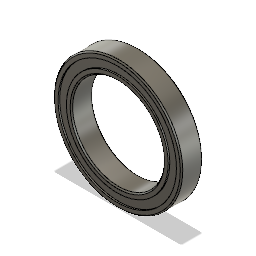
assembly (Autodesk Fusion 360 archive; units mm, degrees)
design "Bearing 42x30x7"
Autodesk Fusion 360 part; units mm, degrees
sketch "Sketch1" plane through (0, 0, 0) normal (0, 1, 0) x (1, 0, 0)
  line L0 (15, 0) -> (15, 3.5)
  line L1 (15, 3.5) -> (16.65, 3.5)
  line L2 (16.65, 3.5) -> (16.65, 3)
  line L3 (16.65, 3) -> (19.35, 3)
  line L4 (19.35, 3) -> (19.35, 3.5)
  line L5 (19.35, 3.5) -> (21, 3.5)
  line L6 (21, 3.5) -> (21, 0)
  line L7 (0, 0) -> (-6, 0) construction
  line L8 (15, 0) -> (15, -3.5)
  line L9 (16.65, -3) -> (19.35, -3)
  line L10 (19.35, -3) -> (19.35, -3.5)
  line L11 (16.65, -3.5) -> (16.65, -3)
  line L12 (15, -3.5) -> (16.65, -3.5)
  line L13 (21, -3.5) -> (21, 0)
  line L14 (19.35, -3.5) -> (21, -3.5)
  line L15 (0, 0) -> (0, 9) construction
  dimension "d3" = 3.5
  dimension "d4" = 3.5
  dimension "d5" = 15
  dimension "d6" = 21
  dimension "d7" = 2.7
  dimension "d8" = 3
  constraint vertical L0
  constraint perpendicular L0 L1
  constraint perpendicular L1 L2
  constraint perpendicular L0 L3
  constraint perpendicular L3 L4
  constraint perpendicular L4 L5
  constraint perpendicular L5 L6
  constraint coincident L7.start L15.start
  constraint parallel L3 L7
  constraint symmetric L0.start L7 L8.start
  constraint symmetric L0.end L7 L8.end
  constraint symmetric L1.end L7 L11.start
  constraint symmetric L2.end L7 L9.start
  constraint symmetric L3.end L7 L9.end
  constraint symmetric L4.end L7 L10.end
  constraint symmetric L5.end L7 L13.start
  constraint symmetric L6.end L7 L13.end
  constraint equal L1 L5
  constraint perpendicular L7 L15
  measures "d3" distance of L7.start L5
  measures "d4" distance of L7.start L1
  measures "d5" distance of L7.start L0
  measures "d6" distance of L7.start L6
  measures "d7" distance of L2.end L3.end
  measures "d8" distance of L7.start L3
revolve "Revolve1" add sketch "Sketch1" angle 360 about axis through (0, 0, 0) along (0, 0, -1)
chamfer "Chamfer1" distance 0.4 angle 45 4 edges at (-19.5789, -7.5939, -3.5) (-13.9849, -5.4242, -3.5) (-19.5789, -7.5939, 3.5) (-13.9849, -5.4242, 3.5)

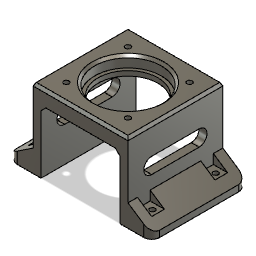
design "bearing_support"
Autodesk Fusion 360 part; units mm, degrees
sketch "Sketch1" plane through (0, 0, 0) normal (0, 0, 1) x (1, 0, 0)
  line L0 (-45, -42) -> (-45, -38)
  line L1 (-45, -38) -> (-30, -38)
  line L2 (-30, -38) -> (-30, 8)
  line L3 (-30, 8) -> (30, 8)
  line L4 (30, 8) -> (30, -38)
  line L5 (30, -38) -> (45, -38)
  line L6 (45, -38) -> (45, -42)
  line L7 (45, -42) -> (25, -42)
  line L8 (25, -42) -> (25, -2)
  line L9 (25, -2) -> (-25, -2)
  line L10 (-25, -2) -> (-25, -42)
  line L11 (-25, -42) -> (-45, -42)
  dimension "d1" = 60
  dimension "d2" = 30
  dimension "d3" = 4
  dimension "d4" = 4
  dimension "d5" = 5
  dimension "d6" = 5
  dimension "d7" = 10
  dimension "d8" = 15
  dimension "d9" = 15
  dimension "d24" = 46
  dimension "d25" = 46
  constraint vertical L0
  constraint perpendicular L0 L1
  constraint perpendicular L1 L2
  constraint perpendicular L2 L3
  constraint perpendicular L3 L4
  constraint perpendicular L4 L5
  constraint perpendicular L5 L6
  constraint perpendicular L6 L7
  constraint perpendicular L7 L8
  constraint perpendicular L8 L9
  constraint perpendicular L9 L10
  constraint perpendicular L0 L11
  measures "d1" distance of L2.end L3.end
  measures "d2" distance of origin L4
  measures "d3" distance of L5.end L6.end
  measures "d4" distance of L0.start L0.end
  measures "d5" distance of L4 L8
  measures "d6" distance of L2 L10
  measures "d7" distance of L3 L9
  measures "d8" distance of L4.end L5.end
  measures "d9" distance of L0.end L1.end
  measures "d24" distance of L3.end L4.end
  measures "d25" distance of L1.end L2.end
extrude "Extrude1" add sketch "Sketch1" along normal blind 60
sketch "Sketch2" plane through (0, 8, 0) normal (0, 1, 0) x (-1, 0, 0)
  line L0 (-30, 0) -> (30, 0)
  line L1 (30, 0) -> (30, 60)
  line L2 (30, 60) -> (-30, 60)
  line L3 (-30, 60) -> (-30, 0)
  circle A0 centre (0, 30) radius 21.1
  dimension "d14" = 42.2
  dimension "d15" = 30
  dimension "d16" = 30
  measures "d14" diameter of A0
  measures "d15" distance of L0 A0.centre
  measures "d16" distance of L3 A0.centre
extrude "Extrude2" cut sketch "Sketch2" against normal blind 7 contours A0
sketch "Sketch3" plane through (0, 1, 0) normal (0, 1, 0) x (-1, 0, 0)
  circle A0 centre (0, 30) radius 21.1
  circle A1 centre (0, 30) radius 19
  dimension "d20" = 38
  constraint concentric A0 A1
  measures "d20" diameter of A1
extrude "Extrude3" cut sketch "Sketch3" against normal up to surface (3 mm away) contours A1
chamfer "Chamfer1" distance 10 distance2 15 1 edges at (-30, -38, 30) measured on face at (-30, -22.6667, 40)
chamfer "Chamfer2" distance 15 distance2 10 1 edges at (30, -38, 30) measured on face at (35, -38, 20)
chamfer "Chamfer3" distance 1.5 angle 45 1 edges at (19.6721, 8, 37.6301)
chamfer "Chamfer4" distance 2 distance2 1 2 edges at (0, 8, 0) (0, 8, 60) measured on face at (33.3323, -36.0007, 0) measured on face at (33.3323, -36.0007, 60)
chamfer "Chamfer5" distance 2 distance2 1 1 edges at (30, 8, 30) measured on face at (30, -5.334, 40)
chamfer "Chamfer6" distance 1 distance2 2 1 edges at (-30, 8, 30) measured on face at (-27.5333, 8, 30)
chamfer "Chamfer7" distance 3 angle 45 2 edges at (25, -2, 30) (-25, -2, 30)
sketch "Sketch4" plane through (0, 8, 0) normal (0, 1, 0) x (-1, 0, 0)
  circle A0 centre (0, 30) radius 22.6
  line L0 (29, 1) -> (29, 59)
  line L1 (29, 59) -> (-29, 59)
  line L2 (-29, 59) -> (-29, 1)
  line L3 (-29, 1) -> (29, 1)
  circle A1 centre (-19.5, 10.5) radius 1.65
  circle A2 centre (19.5, 10.5) radius 1.65
  circle A3 centre (19.5, 49.5) radius 1.65
  circle A4 centre (-19.5, 49.5) radius 1.65
  dimension "d40" = 3.3
  dimension "d41" = 19.5
  dimension "d42" = 19.5
  dimension "d44" = 360
  measures "d40" diameter of A1
  measures "d41" vertical distance of A0.centre A1.centre
  measures "d42" horizontal distance of A0.centre A1.centre
extrude "Extrude4" cut sketch "Sketch4" against normal blind 15 contours A1 | A2 | A3 | A4
sketch "Sketch5" plane through (0, -2, 0) normal (0, -1, 0) x (1, 0, 0)
  circle A0 centre (-19.5, 10.5) radius 1.65
  circle A1 centre (-19.5, 49.5) radius 1.65
  circle A2 centre (19.5, 10.5) radius 1.65
  circle A3 centre (19.5, 49.5) radius 1.65
  circle A4 centre (0, 30) radius 19
  line L0 (-22, 60) -> (-22, 0)
  line L1 (-22, 0) -> (22, 0)
  line L2 (22, 0) -> (22, 60)
  line L3 (22, 60) -> (-22, 60)
  circle A5 centre (19.5, 49.5) radius 4
  circle A6 centre (-19.5, 49.5) radius 4
  circle A7 centre (-19.5, 10.5) radius 4
  circle A8 centre (19.5, 10.5) radius 4
  dimension "d47" = 8
  dimension "d49" = 360
  constraint concentric A3 A5
  measures "d47" diameter of A5
extrude "Extrude5" cut sketch "Sketch5" along normal blind -2 and the other way blind -2 contours L0 A6 | L0 A6 | L2 A5 | L2 A5 | L0 A7 | L0 A7 | L2 A8 | L2 A8
sketch "Sketch6" plane through (0, -42, 0) normal (0, -1, 0) x (1, 0, 0)
  line L0 (25, 0) -> (45, 0)
  line L1 (45, 0) -> (45, 60)
  line L2 (45, 60) -> (25, 60)
  line L3 (25, 60) -> (25, 0)
  circle A0 centre (35.5, 50) radius 1.65
  circle A1 centre (35.5, 10) radius 1.65
  circle A2 centre (-35.5, 10) radius 1.65
  circle A3 centre (-35.5, 50) radius 1.65
  arc A4 (-22, 46.3775) -> (-22, 52.6225) centre (-19.5, 49.5) ccw
  arc A5 (22, 52.6225) -> (22, 46.3775) centre (19.5, 49.5) ccw
  arc A6 (22, 13.6225) -> (22, 7.3775) centre (19.5, 10.5) ccw
  arc A7 (-22, 7.3775) -> (-22, 13.6225) centre (-19.5, 10.5) ccw
  dimension "d54" = 3.3
  dimension "d55" = 10
  dimension "d57" = 3.3
  dimension "d59" = 10
  dimension "d60" = 3.3
  dimension "d61" = 10
  dimension "d63" = 3.3
  dimension "d64" = 10
  dimension "d66" = 16
  dimension "d67" = 16
  dimension "d68" = 16
  dimension "d69" = 16
  measures "d54" diameter of A0
  measures "d55" distance of L2 A0.centre
  measures "d57" diameter of A1
  measures "d59" distance of L0 A1.centre
  measures "d60" diameter of A2
  measures "d61" distance of L0 A2.centre
  measures "d63" diameter of A3
  measures "d64" distance of L2 A3.centre
  measures "d66" horizontal distance of A3.centre A4.centre
  measures "d67" horizontal distance of A0.centre A5.centre
  measures "d68" horizontal distance of A1.centre A6.centre
  measures "d69" horizontal distance of A2.centre A7.centre
extrude "Extrude6" cut sketch "Sketch6" against normal blind 25 contours A0 | A1 | A2 | A3
sketch "Sketch7" plane through (45, 0, 0) normal (1, 0, 0) x (0, 0, -1)
  line L0 (0, -42) -> (0, -38)
  line L1 (0, -38) -> (-60, -38)
  line L2 (-60, -38) -> (-60, -42)
  line L3 (-60, -42) -> (0, -42)
  line L4 (-54, -28) -> (-46, -28)
  line L5 (-46, -28) -> (-46, -34)
  line L6 (-46, -34) -> (-54, -34)
  line L7 (-54, -34) -> (-54, -28)
  line L8 (-14, -28) -> (-6, -28)
  line L9 (-6, -28) -> (-6, -34)
  line L10 (-6, -34) -> (-14, -34)
  line L11 (-14, -34) -> (-14, -28)
  dimension "d72" = 8
  dimension "d73" = 6
  dimension "d74" = 8
  dimension "d75" = 8
  dimension "d76" = 8
  dimension "d77" = 6
  constraint horizontal L4
  constraint vertical L5
  constraint horizontal L6
  constraint vertical L7
  constraint horizontal L8
  constraint vertical L9
  constraint horizontal L10
  constraint vertical L11
  measures "d72" distance of L3 L6
  measures "d73" distance of L4.start L6.end
  measures "d74" distance of L4.start L4.end
  measures "d75" distance of L3 L10
  measures "d76" distance of L8.start L8.end
  measures "d77" distance of L8.end L9.end
extrude "Extrude7" cut sketch "Sketch7" against normal blind 15 contours L4 L5 L6 L7 | L8 L9 L10 L11
sketch "Sketch8" plane through (-45, 0, 0) normal (-1, 0, 0) x (0, 0, 1)
  line L0 (0, -38) -> (0, -42)
  line L1 (0, -42) -> (60, -42)
  line L2 (60, -42) -> (60, -38)
  line L3 (60, -38) -> (0, -38)
  line L4 (6, -28) -> (14, -28)
  line L5 (14, -28) -> (14, -34)
  line L6 (14, -34) -> (6, -34)
  line L7 (6, -34) -> (6, -28)
  line L8 (46, -28) -> (54, -28)
  line L9 (54, -28) -> (54, -34)
  line L10 (54, -34) -> (46, -34)
  line L11 (46, -34) -> (46, -28)
  dimension "d80" = 8
  dimension "d81" = 8
  dimension "d82" = 6
  dimension "d83" = 8
  dimension "d84" = 8
  dimension "d85" = 6
  constraint horizontal L4
  constraint vertical L5
  constraint horizontal L6
  constraint vertical L7
  constraint horizontal L8
  constraint vertical L9
  constraint horizontal L10
  constraint vertical L11
  measures "d80" distance of L1 L6
  measures "d81" distance of L4.start L4.end
  measures "d82" distance of L4.start L6.end
  measures "d83" distance of L1 L10
  measures "d84" distance of L8.start L8.end
  measures "d85" distance of L8.end L9.end
extrude "Extrude8" cut sketch "Sketch8" against normal blind 15 contours L4 L5 L6 L7 | L8 L9 L10 L11
fillet "Fillet1" radius 5 4 edges at (-45, -40, 0) (45, -40, 0) (45, -40, 60) (-45, -40, 60)
sketch "Sketch9" plane through (30, 0, 0) normal (1, 0, 0) x (0, 0, -1)
  line L0 (0, 6) -> (-60, 6)
  line L1 (-60, 6) -> (-60, -28)
  line L2 (-60, -28) -> (-54, -28)
  line L3 (-54, -28) -> (-54, -34)
  line L4 (-54, -34) -> (-46, -34)
  line L5 (-46, -34) -> (-46, -28)
  line L6 (-46, -28) -> (-14, -28)
  line L7 (-14, -28) -> (-14, -34)
  line L8 (-14, -34) -> (-6, -34)
  line L9 (-6, -34) -> (-6, -28)
  line L10 (-6, -28) -> (0, -28)
  line L11 (0, -28) -> (0, 6)
  line L12 (-45, -20) -> (-15, -20)
  arc A0 (-15, -20) -> (-15, -10) centre (-15, -15) ccw
  line L13 (-15, -10) -> (-45, -10)
  arc A1 (-45, -10) -> (-45, -20) centre (-45, -15) ccw
  line L14 (-45, -15) -> (-15, -15) construction
  dimension "d89" = 30
  dimension "d90" = 15
  dimension "d91" = 15
  constraint tangent L12 A0
  constraint tangent A0 L13
  constraint parallel L12 L13
  constraint tangent L13 A1
  constraint tangent L12 A1
  constraint horizontal L14
  measures "d89" distance of A1.centre A0.centre
  measures "d90" distance of L11 A0.centre
  measures "d91" distance of origin L14
extrude "Extrude9" cut sketch "Sketch9" against normal up to surface (60 mm away) contours L12 A0 L13 A1
equation "d1 = main"
equation "d2 = d1 / 2"
equation "d3 = leg_thickness"
equation "d4 = leg_thickness"
equation "d6 = d5"
equation "d8 = leg"
equation "d9 = leg"
equation "main = 60 mm"
equation "d11 = main"
equation "bearing_od = 42.2 mm"
equation "d14 = bearing_od"
equation "d15 = main / 2"
equation "d16 = main / 2"
equation "bearing_thickness = 7 mm"
equation "d18 = -bearing_thickness"
equation "height = 46 mm"
equation "d24 = height"
equation "d25 = height"
equation "leg = 15 mm"
equation "d28 = leg"
equation "d29 = leg"
equation "leg_thickness = 4 mm"
equation "d41 = d42"
equation "d57 = d54"
equation "d59 = d55"
equation "d60 = d54"
equation "d61 = d55"
equation "d63 = d54"
equation "d64 = d55"
equation "d66 = d67"
equation "d68 = d67"
equation "d69 = d67"
equation "d75 = d72"
equation "d76 = d74"
equation "d77 = d73"

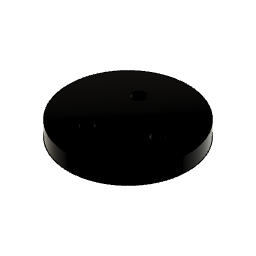
design "bearing_cap"
Autodesk Fusion 360 part; units mm, degrees
sketch "Sketch1" plane through (0, 0, 0) normal (0, 1, 0) x (1, 0, 0)
  circle A0 centre (0, 0) radius 16
  circle A1 centre (8, 0) radius 1.65
  circle A2 centre (-4, 6.9282) radius 1.65
  circle A3 centre (-4, -6.9282) radius 1.65
  dimension "d1" = 32
  dimension "d2" = 3.3
  dimension "d3" = 8
  dimension "d5" = 360
  constraint coincident A0.centre origin
  measures "d1" diameter of A0
  measures "d2" diameter of A1
  measures "d3" distance of A0.centre A1.centre
extrude "Extrude1" add sketch "Sketch1" along normal blind 4

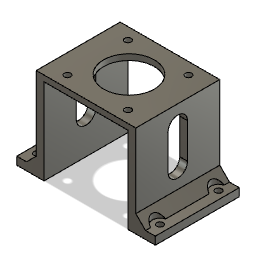
design "motor-support"
Autodesk Fusion 360 part; units mm, degrees
sketch "Sketch1" plane through (0, 0, 0) normal (0, 0, 1) x (1, 0, 0)
  line L0 (-35.5, 0) -> (-21.5, 0)
  line L1 (-21.5, 0) -> (-21.5, 44)
  line L2 (-21.5, 44) -> (21.5, 44)
  line L3 (21.5, 44) -> (21.5, 0)
  line L4 (21.5, 0) -> (35.5, 0)
  line L5 (35.5, 0) -> (35.5, 4)
  line L6 (35.5, 4) -> (25.5, 4)
  line L7 (25.5, 4) -> (25.5, 47)
  line L8 (25.5, 47) -> (-25.5, 47)
  line L9 (-25.5, 47) -> (-25.5, 4)
  line L10 (-25.5, 4) -> (-35.5, 4)
  line L11 (-35.5, 4) -> (-35.5, 0)
  dimension "d1" = 43
  dimension "d2" = 21.5
  dimension "d3" = 4
  dimension "d4" = 4
  dimension "d5" = 3
  dimension "d6" = 4
  dimension "d7" = 4
  dimension "d8" = 10
  dimension "d9" = 10
  dimension "d42" = 44
  dimension "d43" = 44
  constraint horizontal L0
  constraint perpendicular L0 L1
  constraint perpendicular L1 L2
  constraint perpendicular L2 L3
  constraint perpendicular L1 L4
  constraint perpendicular L4 L5
  constraint perpendicular L5 L6
  constraint perpendicular L6 L7
  constraint perpendicular L5 L8
  constraint perpendicular L8 L9
  constraint perpendicular L9 L10
  measures "d1" distance of L1.end L2.end
  measures "d2" distance of origin L3
  measures "d3" distance of L3 L7
  measures "d4" distance of L1 L9
  measures "d5" distance of L2 L8
  measures "d6" distance of L4.end L5.end
  measures "d7" distance of L0 L10
  measures "d8" distance of L5.end L6.end
  measures "d9" distance of L9.end L10.end
  measures "d42" distance of L2.end L3.end
  measures "d43" distance of L0.end L1.end
extrude "Extrude1" add sketch "Sketch1" along normal blind 43
sketch "Sketch3" plane through (0, 44, 0) normal (0, -1, 0) x (1, 0, 0)
  line L0 (-21.5, 0) -> (21.5, 0)
  line L1 (21.5, 0) -> (21.5, 43)
  line L2 (21.5, 43) -> (-21.5, 43)
  line L3 (-21.5, 43) -> (-21.5, 0)
  circle A0 centre (-15.5, 6) radius 1.65
  circle A1 centre (15.5, 6) radius 1.65
  circle A2 centre (-15.5, 37) radius 1.65
  circle A3 centre (15.5, 37) radius 1.65
  dimension "d14" = 3.3
  dimension "d15" = 6
  dimension "d16" = 6
  dimension "d19" = 31
  dimension "d20" = 31
  measures "d14" diameter of A0
  measures "d15" distance of L0 A0.centre
  measures "d16" distance of L3 A0.centre
extrude "Extrude2" cut sketch "Sketch3" against normal up to surface (3 mm away) contours A0 | A1 | A2 | A3
chamfer "Chamfer1" distance 5 angle 45 2 edges at (25.5, 4, 21.5) (-25.5, 4, 21.5)
sketch "Sketch5" plane through (0, 44, 0) normal (0, -1, 0) x (1, 0, 0)
  circle A0 centre (15.5, 37) radius 1.65
  circle A1 centre (15.5, 6) radius 1.65
  circle A2 centre (-15.5, 37) radius 1.65
  circle A3 centre (-15.5, 6) radius 1.65
  line L0 (-21.5, 0) -> (21.5, 0)
  line L1 (21.5, 0) -> (21.5, 43)
  line L2 (21.5, 43) -> (-21.5, 43)
  line L3 (-21.5, 43) -> (-21.5, 0)
  circle A4 centre (0, 21) radius 13
  dimension "d25" = 26
  dimension "d26" = 21.5
  measures "d25" diameter of A4
  measures "d26" distance of L3 A4.centre
extrude "Extrude3" cut sketch "Sketch5" against normal up to surface (3 mm away) contours A4
sketch "Sketch6" plane through (0, 0, 0) normal (0, -1, 0) x (1, 0, 0)
  line L0 (21.5, 0) -> (35.5, 0)
  line L1 (35.5, 0) -> (35.5, 43)
  line L2 (35.5, 43) -> (21.5, 43)
  line L3 (21.5, 43) -> (21.5, 0)
  circle A0 centre (31.5, 36.6) radius 1.65
  circle A1 centre (-31.5, 36.6) radius 1.65
  line L4 (-21.5, 0) -> (-21.5, 43)
  line L5 (-35.5, 43) -> (-21.5, 43)
  circle A2 centre (31.5, 6.6) radius 1.65
  circle A3 centre (-31.5, 6.6) radius 1.65
  dimension "d29" = 3.3
  dimension "d30" = 10
  dimension "d31" = 3.3
  dimension "d32" = 10
  dimension "d33" = 6.4
  dimension "d34" = 6.4
  dimension "d37" = 0
  dimension "d38" = -30
  measures "d29" diameter of A0
  measures "d30" distance of L3 A0.centre
  measures "d31" diameter of A1
  measures "d32" distance of A1.centre L4
  measures "d33" distance of L2 A0.centre
  measures "d34" distance of A1.centre L5
extrude "Extrude4" cut sketch "Sketch6" against normal blind 10 contours A0 | A1 | A2 | A3
sketch "Sketch7" plane through (0, 4, 0) normal (0, 1, 0) x (-1, 0, 0)
  arc A0 (-30.5, 7.9124) -> (-30.5, 5.2876) centre (-31.5, 6.6) ccw
  line L0 (-30.5, 7.9124) -> (-30.5, 35.2876)
  arc A1 (-30.5, 37.9124) -> (-30.5, 35.2876) centre (-31.5, 36.6) ccw
  line L1 (-30.5, 37.9124) -> (-30.5, 43)
  line L2 (-30.5, 43) -> (-35.5, 43)
  line L3 (-35.5, 43) -> (-35.5, 0)
  line L4 (-35.5, 0) -> (-30.5, 0)
  line L5 (-30.5, 0) -> (-30.5, 5.2876)
  circle A2 centre (-31.5, 6.6) radius 4
  circle A3 centre (31.5, 6.6) radius 4
  circle A4 centre (-31.5, 36.6) radius 4
  circle A5 centre (31.5, 36.6) radius 4
  dimension "d44" = 8
  dimension "d47" = 63
  dimension "d48" = 30
  constraint concentric A0 A2
  measures "d44" diameter of A2
extrude "Extrude5" cut sketch "Sketch7" along normal blind 4 contours A0 L0 L5 A2 | A0 L0 L5 A2 | L0 A1 L1 A4 | L0 A1 L1 A4 | A3 | A5
sketch "Sketch8" plane through (25.5, 0, 0) normal (1, 0, 0) x (0, 0, -1)
  line L0 (-43, 9) -> (0, 9)
  line L1 (0, 9) -> (0, 47)
  line L2 (0, 47) -> (-43, 47)
  line L3 (-43, 47) -> (-43, 9)
  line L4 (-26.5, 37) -> (-26.5, 19)
  arc A0 (-26.5, 19) -> (-16.5, 19) centre (-21.5, 19) ccw
  line L5 (-16.5, 19) -> (-16.5, 37)
  arc A1 (-16.5, 37) -> (-26.5, 37) centre (-21.5, 37) ccw
  line L6 (-21.5, 37) -> (-21.5, 19) construction
  dimension "d51" = 18
  dimension "d52" = 10
  dimension "d53" = 21.5
  constraint tangent L4 A0
  constraint tangent A0 L5
  constraint parallel L4 L5
  constraint tangent L5 A1
  constraint tangent L4 A1
  constraint vertical L6
  measures "d51" distance of A1.centre A0.centre
  measures "d52" distance of L2 A1.centre
  measures "d53" distance of L1 A1.centre
extrude "Extrude6" cut sketch "Sketch8" against normal up to surface (51 mm away) contours L4 A0 L5 A1
equation "d1 = size"
equation "d2 = d1 / 2"
equation "d4 = d3"
equation "d7 = d6"
equation "d9 = d8"
equation "d10 = size"
equation "size = 43 mm"
equation "spacing = 31 mm"
equation "d15 = ( size - spacing ) / 2"
equation "d16 = d15"
equation "d26 = size / 2"
equation "d32 = d30"
equation "d34 = d33"
equation "d38 = -( size - 13 mm )"
equation "d43 = d42"
equation "d53 = ( 43 / 2 ) * 1 mm"

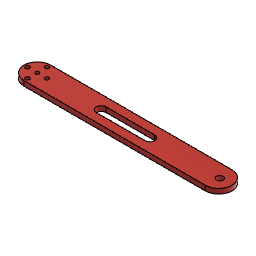
design "pendulum"
Autodesk Fusion 360 part; units mm, degrees
sketch "Sketch1" plane through (0, 0, 0) normal (0, 1, 0) x (1, 0, 0)
  line L0 (-90.5, 11) -> (80.5, 11)
  line L1 (80.5, 11) -> (80.5, -11)
  line L2 (80.5, -11) -> (-90.5, -11)
  line L3 (-90.5, -11) -> (-90.5, 11)
  circle A0 centre (-71.5, 0) radius 1.65
  circle A1 centre (-79.5, 8) radius 1.65
  circle A2 centre (-87.5, 0) radius 1.65
  circle A3 centre (-79.5, -8) radius 1.65
  circle A4 centre (70.5, 0) radius 2.75
  point P0 (-79.5, 0)
  dimension "d6" = 11
  dimension "d7" = 22
  dimension "d10" = 3.3
  dimension "d11" = 8
  dimension "d13" = 360
  dimension "d14" = 5.5
  dimension "d15" = 10
  dimension "d16" = 150
  dimension "d17" = 11
  dimension "d18" = 11
  dimension "d19" = 11
  constraint horizontal L0
  constraint vertical L1
  constraint horizontal L2
  constraint vertical L3
  measures "d6" distance of origin L2
  measures "d7" distance of L0.start L2.end
  measures "d10" diameter of A0
  measures "d11" distance of P0 A0.centre
  measures "d14" diameter of A4
  measures "d15" distance of L1 A4.centre
  measures "d16" distance of P0 A4.centre
  measures "d17" distance of L0 A4.centre
  measures "d18" distance of L0 P0
  measures "d19" distance of L3 P0
extrude "Extrude1" add sketch "Sketch1" along normal blind 4
fillet "Fillet1" radius 11 2 edges at (80.5, 2, -11) (80.5, 2, 11)
fillet "Fillet2" radius 11 2 edges at (-90.5, 2, 11) (-90.5, 2, -11)
sketch "Sketch3" plane through (0, 4, 0) normal (0, 1, 0) x (-1, 0, 0)
  circle A0 centre (79.5, -8) radius 1.65
  circle A1 centre (87.5, 0) radius 1.65
  circle A2 centre (79.5, 8) radius 1.65
  circle A3 centre (-70.5, 0) radius 2.75
  circle A4 centre (71.5, 0) radius 1.65
  arc A5 (79.5, -11) -> (79.5, 11) centre (79.5, 0) ccw
  line L0 (79.5, 11) -> (-69.5, 11)
  arc A6 (-69.5, 11) -> (-69.5, -11) centre (-69.5, 0) ccw
  line L1 (-69.5, -11) -> (79.5, -11)
  line L2 (27, 4) -> (-13, 4)
  arc A7 (-13, 4) -> (-13, -4) centre (-13, 0) ccw
  line L3 (-13, -4) -> (27, -4)
  arc A8 (27, -4) -> (27, 4) centre (27, 0) ccw
  line L4 (27, 0) -> (-13, 0) construction
  dimension "d24" = 8
  dimension "d30" = 40
  constraint tangent L2 A7
  constraint tangent A7 L3
  constraint parallel L2 L3
  constraint tangent L3 A8
  constraint tangent L2 A8
  constraint parallel L1 L4
  measures "d24" diameter of A7
  measures "d30" distance of A8.centre A7.centre
extrude "Extrude2" cut sketch "Sketch3" against normal up to surface (4 mm away) contours L2 A7 L3 A8
sketch "Sketch4" plane through (0, 4, 0) normal (0, 1, 0) x (-1, 0, 0)
  line L0 (27, -4) -> (-13, -4)
  arc A0 (-13, 4) -> (-13, -4) centre (-13, 0) ccw
  line L1 (-13, 4) -> (27, 4)
  arc A1 (27, -4) -> (27, 4) centre (27, 0) ccw
  circle A2 centre (79.5, -8) radius 1.65
  circle A3 centre (87.5, 0) radius 1.65
  circle A4 centre (79.5, 8) radius 1.65
  circle A5 centre (-70.5, 0) radius 2.75
  circle A6 centre (71.5, 0) radius 1.65
  arc A7 (79.5, -11) -> (79.5, 11) centre (79.5, 0) ccw
  line L2 (79.5, 11) -> (-69.5, 11)
  arc A8 (-69.5, 11) -> (-69.5, -11) centre (-69.5, 0) ccw
  line L3 (-69.5, -11) -> (79.5, -11)
  circle A9 centre (79.5, 0) radius 1.5
  dimension "d27" = 3
  constraint concentric A7 A9
  measures "d27" diameter of A9
extrude "Extrude3" cut sketch "Sketch4" against normal up to surface (4 mm away) contours A9
equation "length = 150 mm"
equation "width = 22 mm"
equation "thickness = 4 mm"
equation "d5 = length + width / 2"
equation "d6 = width / 2"
equation "d7 = width"
equation "d16 = length"
equation "d17 = width / 2"
equation "d18 = width / 2"
equation "d20 = thickness"
equation "d22 = width / 2"
equation "d23 = width / 2"

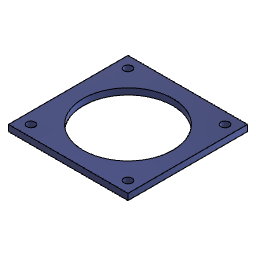
design "bearing_top_cap"
Autodesk Fusion 360 part; units mm, degrees
sketch "Sketch1" plane through (0, 0, 0) normal (0, 1, 0) x (1, 0, 0)
  line L0 (-24, 24) -> (24, 24)
  line L1 (24, 24) -> (24, -24)
  line L2 (24, -24) -> (-24, -24)
  line L3 (-24, -24) -> (-24, 24)
  circle A0 centre (0, 0) radius 18
  circle A1 centre (19.5, -19.5) radius 1.65
  circle A2 centre (19.5, 19.5) radius 1.65
  circle A3 centre (-19.5, 19.5) radius 1.65
  circle A4 centre (-19.5, -19.5) radius 1.65
  dimension "d1" = 24
  dimension "d2" = 48
  dimension "d3" = 24
  dimension "d4" = 48
  dimension "d7" = 36
  dimension "d8" = 3.3
  dimension "d9" = 19.5
  dimension "d10" = 19.5
  dimension "d13" = 360
  constraint horizontal L0
  constraint vertical L1
  constraint horizontal L2
  constraint vertical L3
  constraint coincident A0.centre origin
  measures "d1" distance of A0.centre L0
  measures "d2" distance of L0.start L2.end
  measures "d3" distance of A0.centre L1
  measures "d4" distance of L1.end L2.end
  measures "d7" diameter of A0
  measures "d8" diameter of A1
  measures "d9" horizontal distance of A0.centre A1.centre
  measures "d10" vertical distance of A0.centre A1.centre
extrude "Extrude1" add sketch "Sketch1" along normal blind 2.5
equation "d1 = size / 2"
equation "d2 = size"
equation "d3 = size / 2"
equation "d4 = size"
equation "d9 = ( 39 / 2 ) * 1 mm"
equation "d10 = ( 39 / 2 ) * 1 mm"
equation "size = 48 mm"

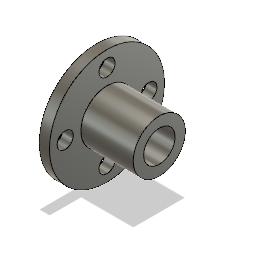
design "Coupler"
Autodesk Fusion 360 part; units mm, degrees
sketch "Sketch1" plane through (0, 0, 0) normal (1, 0, 0) x (0, 0, -1)
  circle A0 centre (0, 0) radius 11
  dimension "d1" = 22
  constraint coincident A0.centre origin
  measures "d1" diameter of A0
extrude "Extrude1" add sketch "Sketch1" along normal blind 2
sketch "Sketch2" plane through (2, 0, 0) normal (1, 0, 0) x (0, 0, -1)
  circle A0 centre (0, 0) radius 11
  circle A1 centre (0, 0) radius 5
  dimension "d4" = 10
  constraint coincident A0.centre A1.centre
  measures "d4" diameter of A1
extrude "Extrude2" add sketch "Sketch2" along normal blind 10 contours A1
sketch "Sketch3" plane through (12, 0, 0) normal (1, 0, 0) x (0, 0, -1)
  circle A0 centre (0, 0) radius 5
  circle A1 centre (0, 0) radius 3
  dimension "d7" = 6
  constraint coincident A0.centre A1.centre
  measures "d7" diameter of A1
extrude "Extrude3" cut sketch "Sketch3" against normal blind 12 contours A1
sketch "Sketch4" plane through (2, 0, 0) normal (1, 0, 0) x (0, 0, -1)
  circle A0 centre (0, 0) radius 5
  circle A1 centre (0, 0) radius 11
  circle A2 centre (8, 0) radius 1.55
  circle A3 centre (0, 8) radius 1.55
  circle A4 centre (-8, 0) radius 1.55
  circle A5 centre (0, -8) radius 1.55
  dimension "d10" = 3.1
  dimension "d11" = 8
  dimension "d13" = 360
  measures "d10" diameter of A2
  measures "d11" distance of A0.centre A2.centre
extrude "Extrude4" cut sketch "Sketch4" against normal up to surface (2 mm away) contours A2 | A3 | A4 | A5

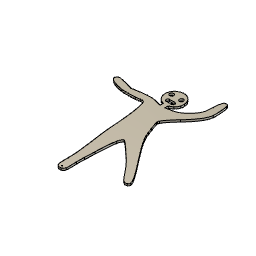
design "human"
Autodesk Fusion 360 part; units mm, degrees
sketch "Sketch1" plane through (0, 0, 0) normal (0, 1, 0) x (1, 0, 0)
  spline S0 degree 3 poles (28.5505, 138.7144) (26.7377, 138.2108) (26.0126, 135.8139) (25.6097, 128.7641) knots 0 0 0 0 1 1 1 1
  spline S1 degree 3 poles (25.6097, 128.7641) (25.1062, 119.7605) (24.5019, 117.988) (20.3324, 113.3552) knots 0 0 0 0 1 1 1 1
  spline S2 degree 3 poles (20.3324, 113.3552) (14.6322, 107.0104) (12.2151, 105.7213) (3.1309, 104.1703) knots 0 0 0 0 1 1 1 1
  spline S3 degree 3 poles (3.1309, 104.1703) (-1.1191, 103.4654) (-3.1132, 103.4654) (-5.5101, 104.1905) knots 0 0 0 0 1 1 1 1
  spline S4 degree 3 poles (-5.5101, 104.1905) (-13.4462, 106.6277) (-16.2057, 106.668) (-28.8752, 104.5732) knots 0 0 0 0 1 1 1 1
  line L0 (-28.8752, 104.5732) -> (-33.3267, 103.8481)
  line L1 (-33.3267, 103.8481) -> (-36.8314, 104.8552)
  spline S5 degree 3 poles (-36.8314, 104.8552) (-44.1632, 106.9701) (-47.4061, 107.6348) (-49.1182, 107.3931) knots 0 0 0 0 1 1 1 1
  spline S6 degree 3 poles (-49.1182, 107.3931) (-50.9915, 107.1111) (-51.918, 105.1775) (-50.931, 103.6064) knots 0 0 0 0 1 1 1 1
  spline S7 degree 3 poles (-50.931, 103.6064) (-49.6218, 101.4713) (-43.5388, 99.0945) (-37.2343, 98.2284) knots 0 0 0 0 1 1 1 1
  spline S8 degree 3 poles (-37.2343, 98.2284) (-34.5956, 97.8658) (-26.9818, 97.9262) (-23.4368, 98.3291) knots 0 0 0 0 1 1 1 1
  spline S9 degree 3 poles (-23.4368, 98.3291) (-21.8858, 98.4902) (-19.6702, 98.7521) (-18.5019, 98.8729) knots 0 0 0 0 1 1 1 1
  spline S10 degree 3 poles (-18.5019, 98.8729) (-15.259, 99.2556) (-15.1986, 99.2153) (-14.1915, 96.1336) knots 0 0 0 0 1 1 1 1
  spline S11 degree 3 poles (-14.1915, 96.1336) (-12.3384, 90.4534) (-10.6464, 78.8917) (-9.74, 65.618) knots 0 0 0 0 1 1 1 1
  spline S12 degree 3 poles (-9.74, 65.618) (-9.1358, 56.8762) (-8.3502, 49.6048) (-7.1215, 41.3465) knots 0 0 0 0 1 1 1 1
  spline S13 degree 3 poles (-7.1215, 41.3465) (-6.5173, 37.318) (-5.7518, 31.4365) (-4.4829, 20.902) knots 0 0 0 0 1 1 1 1
  spline S14 degree 3 poles (-4.4829, 20.902) (-4.2613, 19.049) (-4.1002, 15.5039) (-3.9995, 9.8238) knots 0 0 0 0 1 1 1 1
  spline S15 degree 3 poles (-3.9995, 9.8238) (-3.8383, 0.3972) (-3.7779, -0.1265) (-2.4082, -1.4761) knots 0 0 0 0 1 1 1 1
  spline S16 degree 3 poles (-2.4082, -1.4761) (-1.5018, -2.3825) (-0.2933, -2.6443) (1.3584, -2.2818) knots 0 0 0 0 1 1 1 1
  spline S17 degree 3 poles (1.3584, -2.2818) (2.7079, -1.9796) (3.4935, -1.1336) (3.856, 0.377) knots 0 0 0 0 1 1 1 1
  spline S18 degree 3 poles (3.856, 0.377) (4.1582, 1.5856) (4.1783, 5.2515) (3.9567, 10.7302) knots 0 0 0 0 1 1 1 1
  spline S19 degree 3 poles (3.9567, 10.7302) (3.8762, 12.6638) (3.9165, 16.3096) (4.0373, 19.0087) knots 0 0 0 0 1 1 1 1
  spline S20 degree 3 poles (4.0373, 19.0087) (4.1582, 21.6473) (4.3596, 26.2196) (4.4603, 29.1604) knots 0 0 0 0 1 1 1 1
  spline S21 degree 3 poles (4.4603, 29.1604) (4.8631, 38.9093) (5.4674, 46.2008) (6.1925, 49.6451) knots 0 0 0 0 1 1 1 1
  spline S22 degree 3 poles (6.1925, 49.6451) (6.8371, 52.747) (7.8442, 54.5397) (8.952, 54.5397) knots 0 0 0 0 1 1 1 1
  spline S23 degree 3 poles (8.952, 54.5397) (9.7174, 54.5397) (13.9876, 50.8738) (22.4272, 42.9176) knots 0 0 0 0 1 1 1 1
  spline S24 degree 3 poles (22.4272, 42.9176) (30.464, 35.3441) (34.0494, 31.4365) (39.9108, 23.9234) knots 0 0 0 0 1 1 1 1
  spline S25 degree 3 poles (39.9108, 23.9234) (44.8255, 17.5987) (46.6383, 16.37) (49.1158, 17.639) knots 0 0 0 0 1 1 1 1
  spline S26 degree 3 poles (49.1158, 17.639) (50.1833, 18.203) (50.4653, 18.7065) (50.3042, 19.8345) knots 0 0 0 0 1 1 1 1
  spline S27 degree 3 poles (50.3042, 19.8345) (49.9013, 22.7954) (46.3362, 28.113) (34.7745, 43.0586) knots 0 0 0 0 1 1 1 1
  spline S28 degree 3 poles (34.7745, 43.0586) (22.5682, 58.8099) (18.2981, 65.054) (15.8407, 70.6535) knots 0 0 0 0 1 1 1 1
  spline S29 degree 3 poles (15.8407, 70.6535) (13.8265, 75.2863) (10.6641, 83.8065) (9.9793, 86.4854) knots 0 0 0 0 1 1 1 1
  line L2 (9.9793, 86.4854) -> (9.6167, 87.8954)
  line L3 (9.6167, 87.8954) -> (10.2411, 89.2046)
  spline S30 degree 3 poles (10.2411, 89.2046) (11.349, 91.5411) (14.3905, 95.3883) (19.849, 101.2497) knots 0 0 0 0 1 1 1 1
  spline S31 degree 3 poles (19.849, 101.2497) (28.4699, 110.5555) (31.9143, 116.0543) (32.6797, 121.7546) knots 0 0 0 0 1 1 1 1
  spline S32 degree 3 poles (32.6797, 121.7546) (33.0825, 124.8565) (32.5387, 133.1148) (31.6726, 136.4987) knots 0 0 0 0 1 1 1 1
  spline S33 degree 3 poles (31.6726, 136.4987) (31.451, 137.4051) (31.2093, 137.9087) (30.8467, 138.1706) knots 0 0 0 0 1 1 1 1
  spline S34 degree 3 poles (30.8467, 138.1706) (30.1417, 138.6741) (29.2353, 138.8957) (28.5505, 138.7144) knots 0 0 0 0 1 1 1 1
  spline S35 degree 3 poles (-3.9793, 125.924) (-6.5173, 125.2392) (-9.1156, 123.1645) (-10.2234, 120.9287) knots 0 0 0 0 1 1 1 1
  spline S36 degree 3 poles (-10.2234, 120.9287) (-12.8419, 115.591) (-10.2637, 109.2261) (-4.7246, 107.3125) knots 0 0 0 0 1 1 1 1
  spline S37 degree 3 poles (-4.7246, 107.3125) (-1.2803, 106.1241) (2.3856, 106.9097) (5.0243, 109.4073) knots 0 0 0 0 1 1 1 1
  spline S38 degree 3 poles (5.0243, 109.4073) (6.394, 110.6763) (7.1392, 111.8244) (7.7032, 113.4962) knots 0 0 0 0 1 1 1 1
  spline S39 degree 3 poles (7.7032, 113.4962) (8.0658, 114.5839) (8.1262, 115.1479) (8.0456, 116.9406) knots 0 0 0 0 1 1 1 1
  spline S40 degree 3 poles (8.0456, 116.9406) (7.9852, 118.9347) (7.9248, 119.2166) (7.1997, 120.6669) knots 0 0 0 0 1 1 1 1
  spline S41 degree 3 poles (7.1997, 120.6669) (5.1653, 124.8766) (0.4117, 127.1124) (-3.9793, 125.924) knots 0 0 0 0 1 1 1 1
  line L4 (1.3199, 107.2081) -> (1.3199, 103.8951)
  line L5 (-3.5162, 106.9777) -> (-3.5162, 103.7492)
  circle A0 centre (3, 119) radius 2
  circle A1 centre (-7, 119) radius 2
  line L6 (-4, 110.2788) -> (1.4991, 110.2788)
  arc A2 (1.4991, 110.2788) -> (1.4991, 113.7212) centre (1.4991, 112) ccw
  line L7 (1.4991, 113.7212) -> (-4, 113.7212)
  arc A3 (-4, 113.7212) -> (-4, 110.2788) centre (-4, 112) ccw
  line L8 (-4, 112) -> (1.4991, 112) construction
  dimension "d1" = 4
  dimension "d2" = 4
  constraint coincident S37 L4.start
  constraint coincident S3 L4.end
  constraint vertical L4
  constraint coincident S37 L5.start
  constraint coincident S3 L5.end
  constraint parallel L4 L5
  constraint tangent L6 A2
  constraint tangent A2 L7
  constraint parallel L6 L7
  constraint tangent L7 A3
  constraint tangent L6 A3
  constraint horizontal L8
  measures "d1" diameter of A0
  measures "d2" diameter of A1
extrude "Extrude1" add sketch "Sketch1" along normal blind 2
sketch "Sketch2" plane through (0, 2, 0) normal (0, 1, 0) x (-1, 0, 0)
  arc A0 (4, -113.7212) -> (4, -110.2788) centre (4, -112) ccw
  line L0 (4, -113.7212) -> (-1.4991, -113.7212)
  arc A1 (-1.4991, -110.2788) -> (-1.4991, -113.7212) centre (-1.4991, -112) ccw
  line L1 (-1.4991, -110.2788) -> (4, -110.2788)
  circle A2 centre (-3, -119) radius 2
  circle A3 centre (7, -119) radius 2
  spline S0 degree 3 poles (-1.3199, -107.2081) (-2.6712, -107.6373) (-3.9352, -108.3765) (-5.0243, -109.4073) knots 0.587264 0.587264 0.587264 0.587264 1 1 1 1
  spline S1 degree 3 poles (-5.0243, -109.4073) (-6.394, -110.6763) (-7.1392, -111.8244) (-7.7032, -113.4962) knots 0 0 0 0 1 1 1 1
  spline S2 degree 3 poles (-7.7032, -113.4962) (-8.0658, -114.5839) (-8.1262, -115.1479) (-8.0456, -116.9406) knots 0 0 0 0 1 1 1 1
  spline S3 degree 3 poles (-8.0456, -116.9406) (-7.9852, -118.9347) (-7.9248, -119.2166) (-7.1997, -120.6669) knots 0 0 0 0 1 1 1 1
  spline S4 degree 3 poles (-7.1997, -120.6669) (-5.1653, -124.8766) (-0.4117, -127.1124) (3.9793, -125.924) knots 0 0 0 0 1 1 1 1
  spline S5 degree 3 poles (3.9793, -125.924) (6.5173, -125.2392) (9.1156, -123.1645) (10.2234, -120.9287) knots 0 0 0 0 1 1 1 1
  spline S6 degree 3 poles (10.2234, -120.9287) (12.8419, -115.591) (10.2637, -109.2261) (4.7246, -107.3125) knots 0 0 0 0 1 1 1 1
  spline S7 degree 3 poles (4.7246, -107.3125) (4.3241, -107.1744) (3.9207, -107.0629) (3.5162, -106.9777) knots 0 0 0 0 0.116263 0.116263 0.116263 0.116263
  line L2 (3.5162, -106.9777) -> (3.5162, -103.7492)
  spline S8 degree 3 poles (3.5162, -103.7492) (4.1886, -103.8388) (4.8333, -103.9857) (5.5101, -104.1905) knots 0.717636 0.717636 0.717636 0.717636 1 1 1 1
  spline S9 degree 3 poles (5.5101, -104.1905) (13.4462, -106.6277) (16.2057, -106.668) (28.8752, -104.5732) knots 0 0 0 0 1 1 1 1
  line L3 (28.8752, -104.5732) -> (33.3267, -103.8481)
  line L4 (33.3267, -103.8481) -> (36.8314, -104.8552)
  spline S10 degree 3 poles (36.8314, -104.8552) (44.1632, -106.9701) (47.4061, -107.6348) (49.1182, -107.3931) knots 0 0 0 0 1 1 1 1
  spline S11 degree 3 poles (49.1182, -107.3931) (50.9915, -107.1111) (51.918, -105.1775) (50.931, -103.6064) knots 0 0 0 0 1 1 1 1
  spline S12 degree 3 poles (50.931, -103.6064) (49.6218, -101.4713) (43.5388, -99.0945) (37.2343, -98.2284) knots 0 0 0 0 1 1 1 1
  spline S13 degree 3 poles (37.2343, -98.2284) (34.5956, -97.8658) (26.9818, -97.9262) (23.4368, -98.3291) knots 0 0 0 0 1 1 1 1
  spline S14 degree 3 poles (23.4368, -98.3291) (21.8858, -98.4902) (19.6702, -98.7521) (18.5019, -98.8729) knots 0 0 0 0 1 1 1 1
  spline S15 degree 3 poles (18.5019, -98.8729) (15.259, -99.2556) (15.1986, -99.2153) (14.1915, -96.1336) knots 0 0 0 0 1 1 1 1
  spline S16 degree 3 poles (14.1915, -96.1336) (12.3384, -90.4534) (10.6464, -78.8917) (9.74, -65.618) knots 0 0 0 0 1 1 1 1
  spline S17 degree 3 poles (9.74, -65.618) (9.1358, -56.8762) (8.3502, -49.6048) (7.1215, -41.3465) knots 0 0 0 0 1 1 1 1
  spline S18 degree 3 poles (7.1215, -41.3465) (6.5173, -37.318) (5.7518, -31.4365) (4.4829, -20.902) knots 0 0 0 0 1 1 1 1
  spline S19 degree 3 poles (4.4829, -20.902) (4.2613, -19.049) (4.1002, -15.5039) (3.9995, -9.8238) knots 0 0 0 0 1 1 1 1
  spline S20 degree 3 poles (3.9995, -9.8238) (3.8383, -0.3972) (3.7779, 0.1265) (2.4082, 1.4761) knots 0 0 0 0 1 1 1 1
  spline S21 degree 3 poles (2.4082, 1.4761) (1.5018, 2.3825) (0.2933, 2.6443) (-1.3584, 2.2818) knots 0 0 0 0 1 1 1 1
  spline S22 degree 3 poles (-1.3584, 2.2818) (-2.7079, 1.9796) (-3.4935, 1.1336) (-3.856, -0.377) knots 0 0 0 0 1 1 1 1
  spline S23 degree 3 poles (-3.856, -0.377) (-4.1582, -1.5856) (-4.1783, -5.2515) (-3.9567, -10.7302) knots 0 0 0 0 1 1 1 1
  spline S24 degree 3 poles (-3.9567, -10.7302) (-3.8762, -12.6638) (-3.9165, -16.3096) (-4.0373, -19.0087) knots 0 0 0 0 1 1 1 1
  spline S25 degree 3 poles (-4.0373, -19.0087) (-4.1582, -21.6473) (-4.3596, -26.2196) (-4.4603, -29.1604) knots 0 0 0 0 1 1 1 1
  spline S26 degree 3 poles (-4.4603, -29.1604) (-4.8631, -38.9093) (-5.4674, -46.2008) (-6.1925, -49.6451) knots 0 0 0 0 1 1 1 1
  spline S27 degree 3 poles (-6.1925, -49.6451) (-6.8371, -52.747) (-7.8442, -54.5397) (-8.952, -54.5397) knots 0 0 0 0 1 1 1 1
  spline S28 degree 3 poles (-8.952, -54.5397) (-9.7174, -54.5397) (-13.9876, -50.8738) (-22.4272, -42.9176) knots 0 0 0 0 1 1 1 1
  spline S29 degree 3 poles (-22.4272, -42.9176) (-30.464, -35.3441) (-34.0494, -31.4365) (-39.9108, -23.9234) knots 0 0 0 0 1 1 1 1
  spline S30 degree 3 poles (-39.9108, -23.9234) (-44.8255, -17.5987) (-46.6383, -16.37) (-49.1158, -17.639) knots 0 0 0 0 1 1 1 1
  spline S31 degree 3 poles (-49.1158, -17.639) (-50.1833, -18.203) (-50.4653, -18.7065) (-50.3042, -19.8345) knots 0 0 0 0 1 1 1 1
  spline S32 degree 3 poles (-50.3042, -19.8345) (-49.9013, -22.7954) (-46.3362, -28.113) (-34.7745, -43.0586) knots 0 0 0 0 1 1 1 1
  spline S33 degree 3 poles (-34.7745, -43.0586) (-22.5682, -58.8099) (-18.2981, -65.054) (-15.8407, -70.6535) knots 0 0 0 0 1 1 1 1
  spline S34 degree 3 poles (-15.8407, -70.6535) (-13.8265, -75.2863) (-10.6641, -83.8065) (-9.9793, -86.4854) knots 0 0 0 0 1 1 1 1
  line L5 (-9.9793, -86.4854) -> (-9.6167, -87.8954)
  line L6 (-9.6167, -87.8954) -> (-10.2411, -89.2046)
  spline S35 degree 3 poles (-10.2411, -89.2046) (-11.349, -91.5411) (-14.3905, -95.3883) (-19.849, -101.2497) knots 0 0 0 0 1 1 1 1
  spline S36 degree 3 poles (-19.849, -101.2497) (-28.4699, -110.5555) (-31.9143, -116.0543) (-32.6797, -121.7546) knots 0 0 0 0 1 1 1 1
  spline S37 degree 3 poles (-32.6797, -121.7546) (-33.0825, -124.8565) (-32.5387, -133.1148) (-31.6726, -136.4987) knots 0 0 0 0 1 1 1 1
  spline S38 degree 3 poles (-31.6726, -136.4987) (-31.451, -137.4051) (-31.2093, -137.9087) (-30.8467, -138.1706) knots 0 0 0 0 1 1 1 1
  spline S39 degree 3 poles (-30.8467, -138.1706) (-30.1417, -138.6741) (-29.2353, -138.8957) (-28.5505, -138.7144) knots 0 0 0 0 1 1 1 1
  spline S40 degree 3 poles (-28.5505, -138.7144) (-26.7377, -138.2108) (-26.0126, -135.8139) (-25.6097, -128.7641) knots 0 0 0 0 1 1 1 1
  spline S41 degree 3 poles (-25.6097, -128.7641) (-25.1062, -119.7605) (-24.5019, -117.988) (-20.3324, -113.3552) knots 0 0 0 0 1 1 1 1
  spline S42 degree 3 poles (-20.3324, -113.3552) (-14.6322, -107.0104) (-12.2151, -105.7213) (-3.1309, -104.1703) knots 0 0 0 0 1 1 1 1
  spline S43 degree 3 poles (-3.1309, -104.1703) (-2.4771, -104.0619) (-1.8767, -103.9701) (-1.3199, -103.8951) knots 0 0 0 0 0.15384 0.15384 0.15384 0.15384
  line L7 (-1.3199, -103.8951) -> (-1.3199, -107.2081)
  circle A4 centre (0, 0) radius 0.5
  dimension "d5" = 1
  constraint coincident A4.centre origin
  measures "d5" diameter of A4
extrude "Extrude2" cut sketch "Sketch2" against normal up to surface (2 mm away) contours A4

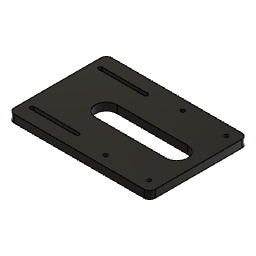
design "base"
Autodesk Fusion 360 part; units mm, degrees
sketch "Sketch1" plane through (0, 0, 0) normal (0, 1, 0) x (1, 0, 0)
  line L0 (-65, 45) -> (65, 45)
  line L1 (65, 45) -> (65, -45)
  line L2 (65, -45) -> (-65, -45)
  line L3 (-65, -45) -> (-65, 45)
  circle A0 centre (55, 35.5) radius 1.65
  circle A1 centre (15, 35.5) radius 1.65
  circle A2 centre (55, -35.5) radius 1.65
  circle A3 centre (15, -35.5) radius 1.65
  dimension "d4" = 65
  dimension "d5" = 45
  dimension "d8" = 90
  dimension "d9" = 130
  dimension "d10" = 3.3
  dimension "d12" = 10
  dimension "d13" = 9.5
  dimension "d16" = -40
  dimension "d17" = -71
  constraint horizontal L0
  constraint vertical L1
  constraint horizontal L2
  constraint vertical L3
  measures "d4" distance of origin L3
  measures "d5" distance of origin L2
  measures "d8" distance of L0.end L1.end
  measures "d9" distance of L0.start L0.end
  measures "d10" diameter of A0
  measures "d12" distance of L1 A0.centre
  measures "d13" distance of L0 A0.centre
extrude "Extrude1" add sketch "Sketch1" along normal blind 7
sketch "Sketch2" plane through (0, 7, 0) normal (0, 1, 0) x (-1, 0, 0)
  circle A0 centre (-55, 35.5) radius 1.65
  circle A1 centre (-15, 35.5) radius 1.65
  circle A2 centre (-15, -35.5) radius 1.65
  circle A3 centre (-55, -35.5) radius 1.65
  line L0 (65, 45) -> (-65, 45)
  line L1 (-65, 45) -> (-65, -45)
  line L2 (-65, -45) -> (65, -45)
  line L3 (65, -45) -> (65, 45)
  line L4 (-45, -10) -> (20, -10)
  arc A4 (20, -10) -> (20, 10) centre (20, 0) ccw
  line L5 (20, 10) -> (-45, 10)
  arc A5 (-45, 10) -> (-45, -10) centre (-45, 0) ccw
  line L6 (-45, 0) -> (20, 0) construction
  dimension "d18" = 65
  dimension "d19" = 20
  dimension "d20" = 10
  dimension "d22" = 45
  constraint tangent L4 A4
  constraint tangent A4 L5
  constraint parallel L4 L5
  constraint tangent L5 A5
  constraint tangent L4 A5
  constraint horizontal L6
  measures "d18" distance of A5.centre A4.centre
  measures "d19" distance of L1 A5.centre
  measures "d20" radius of A5
  measures "d22" distance of L0 L6
extrude "Extrude2" cut sketch "Sketch2" against normal up to surface (7 mm away) contours L4 A4 L5 A5
fillet "Fillet1" radius 5 4 edges at (65, 3.5, 45) (-65, 3.5, 45) (-65, 3.5, -45) (65, 3.5, -45)
sketch "Sketch3" plane through (0, 7, 0) normal (0, 1, 0) x (-1, 0, 0)
  arc A0 (-65, -40) -> (-60, -45) centre (-60, -40) ccw
  line L0 (-60, -45) -> (60, -45)
  arc A1 (60, -45) -> (65, -40) centre (60, -40) ccw
  line L1 (65, -40) -> (65, 40)
  arc A2 (65, 40) -> (60, 45) centre (60, 40) ccw
  line L2 (60, 45) -> (-60, 45)
  arc A3 (-60, 45) -> (-65, 40) centre (-60, 40) ccw
  line L3 (-65, 40) -> (-65, -40)
  line L4 (-45, 10) -> (20, 10)
  arc A4 (20, -10) -> (20, 10) centre (20, 0) ccw
  line L5 (20, -10) -> (-45, -10)
  arc A5 (-45, 10) -> (-45, -10) centre (-45, 0) ccw
  circle A6 centre (-55, 35.5) radius 1.65
  circle A7 centre (-15, 35.5) radius 1.65
  circle A8 centre (-15, -35.5) radius 1.65
  circle A9 centre (-55, -35.5) radius 1.65
  line L6 (57, -29.85) -> (15, -29.85)
  arc A10 (15, -29.85) -> (15, -33.15) centre (15, -31.5) ccw
  line L7 (15, -33.15) -> (57, -33.15)
  arc A11 (57, -33.15) -> (57, -29.85) centre (57, -31.5) ccw
  line L8 (57, -31.5) -> (15, -31.5) construction
  line L9 (0, 0) -> (102, 0) construction
  arc A12 (15, 33.15) -> (15, 29.85) centre (15, 31.5) ccw
  line L10 (15, 33.15) -> (57, 33.15)
  line L11 (57, 29.85) -> (15, 29.85)
  arc A13 (57, 29.85) -> (57, 33.15) centre (57, 31.5) ccw
  dimension "d26" = 3.3
  dimension "d27" = 8
  dimension "d28" = 42
  dimension "d30" = 31.5
  constraint tangent L6 A10
  constraint tangent A10 L7
  constraint parallel L6 L7
  constraint tangent L7 A11
  constraint tangent L6 A11
  constraint horizontal L8
  constraint coincident L9.start origin
  constraint horizontal L9
  constraint symmetric L6.start L9 L11.start
  constraint symmetric L6.end L9 A12.end
  constraint symmetric A10.end L9 A12.start
  constraint symmetric L7.end L9 L10.end
  constraint symmetric A10 L9 A12
  constraint symmetric A11 L9 A13
  measures "d26" diameter of A10
  measures "d27" distance of L1 A11.centre
  measures "d28" distance of A11.centre A10.centre
  measures "d30" distance of L8 L9
extrude "Extrude3" cut sketch "Sketch3" against normal up to surface (7 mm away) contours L6 A10 L7 A11 | A12 L10 L11 A13
sketch "Sketch4" plane through (0, 0, 0) normal (0, -1, 0) x (1, 0, 0)
  line L0 (-15, -33.15) -> (-57, -33.15)
  arc A0 (-57, -29.85) -> (-57, -33.15) centre (-57, -31.5) ccw
  line L1 (-57, -29.85) -> (-15, -29.85)
  arc A1 (-15, -33.15) -> (-15, -29.85) centre (-15, -31.5) ccw
  line L2 (-57, 33.15) -> (-15, 33.15)
  arc A2 (-15, 29.85) -> (-15, 33.15) centre (-15, 31.5) ccw
  line L3 (-15, 29.85) -> (-57, 29.85)
  arc A3 (-57, 33.15) -> (-57, 29.85) centre (-57, 31.5) ccw
  line L4 (-20, 10) -> (45, 10)
  arc A4 (45, -10) -> (45, 10) centre (45, 0) ccw
  line L5 (45, -10) -> (-20, -10)
  arc A5 (-20, 10) -> (-20, -10) centre (-20, 0) ccw
  circle A6 centre (55, 35.5) radius 1.65
  circle A7 centre (15, 35.5) radius 1.65
  circle A8 centre (15, -35.5) radius 1.65
  circle A9 centre (55, -35.5) radius 1.65
  arc A10 (60, -45) -> (65, -40) centre (60, -40) ccw
  line L6 (65, -40) -> (65, 40)
  arc A11 (65, 40) -> (60, 45) centre (60, 40) ccw
  line L7 (60, 45) -> (-60, 45)
  arc A12 (-60, 45) -> (-65, 40) centre (-60, 40) ccw
  line L8 (-65, 40) -> (-65, -40)
  arc A13 (-65, -40) -> (-60, -45) centre (-60, -40) ccw
  line L9 (-60, -45) -> (60, -45)
  circle A14 centre (55, 35.5) radius 4
  circle A15 centre (55, -35.5) radius 4
  circle A16 centre (15, 35.5) radius 4
  circle A17 centre (15, -35.5) radius 4
  line L10 (-57, 27.5) -> (-15, 27.5)
  arc A18 (-15, 27.5) -> (-15, 35.5) centre (-15, 31.5) ccw
  line L11 (-15, 35.5) -> (-57, 35.5)
  arc A19 (-57, 35.5) -> (-57, 27.5) centre (-57, 31.5) ccw
  line L12 (-57, 31.5) -> (-15, 31.5) construction
  line L13 (-57, -35.5) -> (-15, -35.5)
  arc A20 (-15, -35.5) -> (-15, -27.5) centre (-15, -31.5) ccw
  line L14 (-15, -27.5) -> (-57, -27.5)
  arc A21 (-57, -27.5) -> (-57, -35.5) centre (-57, -31.5) ccw
  line L15 (-57, -31.5) -> (-15, -31.5) construction
  dimension "d33" = 8
  dimension "d34" = 8
  dimension "d35" = 8
  dimension "d36" = 8
  dimension "d37" = 8
  dimension "d38" = 8
  constraint concentric A6 A14
  constraint concentric A9 A15
  constraint concentric A7 A16
  constraint concentric A8 A17
  constraint tangent L10 A18
  constraint tangent A18 L11
  constraint parallel L10 L11
  constraint tangent L11 A19
  constraint tangent L10 A19
  constraint coincident A2.centre A18.centre
  constraint parallel L3 L12
  constraint coincident A3.centre A19.centre
  constraint tangent L13 A20
  constraint tangent A20 L14
  constraint parallel L13 L14
  constraint tangent L14 A21
  constraint tangent L13 A21
  constraint coincident A1.centre A20.centre
  constraint parallel L0 L15
  constraint coincident A0.centre A21.centre
  measures "d33" diameter of A14
  measures "d34" diameter of A15
  measures "d35" diameter of A16
  measures "d36" diameter of A17
  measures "d37" diameter of A18
  measures "d38" diameter of A20
extrude "Extrude4" cut sketch "Sketch4" against normal blind 3 contours A14 | A15 | A16 | A17 | L10 A18 L11 A19 | L13 A20 L14 A21
equation "length = 130 mm"
equation "width = 90 mm"
equation "thickness = 7 mm"
equation "d4 = length / 2"
equation "d5 = width / 2"
equation "d6 = thickness"
equation "d8 = width"
equation "d9 = length"
equation "d10 = d11"
equation "d11 = 3.3 mm"
equation "d13 = ( width - 71 mm ) / 2"
equation "d22 = width / 2"
equation "d30 = ( 63 / 2 ) * 1 mm"
